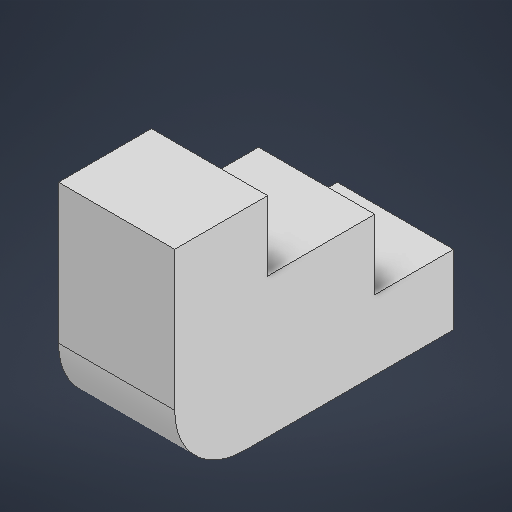
# Autodesk Inventor part: Part4
Saved by Autodesk Inventor 2026 (Build 300175050, 175E)
## iProperties
Created: 2026-03-19
Part Number: Part4
Material: Generic
Document SubType Name: Modeling
Designer: Administrator
Density: 1 g/cm^3
Appearance: Default
Author: Administrator
Autodesk Inventor part; units mm, degrees
ref_plane "YZ Plane" through (0, 0, 0) normal (1, 0, 0) x (0, 1, 0)
ref_plane "XZ Plane" through (0, 0, 0) normal (0, 1, 0) x (-1, 0, 0)
ref_plane "XY Plane" through (0, 0, 0) normal (0, 0, 1) x (1, 0, 0)
sketch "Sketch1" plane through (0, 0, 0) normal (1, 0, 0) x (0, 1, 0)
  line L0 (0, 0) -> (0, -60)
  line L1 (0, -60) -> (15, -60)
  line L2 (15, -60) -> (15, -43.0556)
  line L3 (15, -43.0556) -> (30, -43.0556)
  line L4 (30, -43.0556) -> (30, -20)
  line L5 (30, -20) -> (45, -20)
  line L6 (45, -20) -> (45, 0)
  line L7 (45, 0) -> (0, 0)
  dimension "d0" = 15
  dimension "d1" = 15
  dimension "d2" = 20
  dimension "d3" = 45
  dimension "d4" = 60
  constraints: 16 end point, 7 perpendicular, 1 vertical
  measures "d0" distance of L2.end L3.end
  measures "d1" distance of L0.end L1.end
  measures "d2" distance of L5.end L6.end
  measures "d3" distance of L6.end L0.start
  measures "d4" distance of L0.start L0.end
extrude "Extrusion1" add sketch "Sketch1" along normal blind 25
fillet "Fillet1" radius 15 1 edges at (12.5, 0, 0)
body "Solid1"
